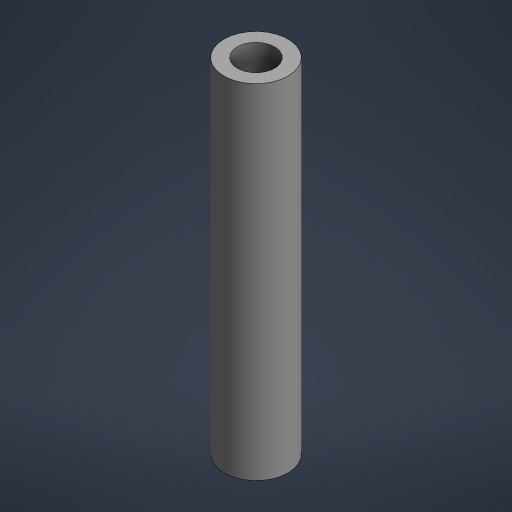
# Autodesk Inventor part: PDP_Spacer
Saved by Autodesk Inventor 2023 (Build 270158000, 158)
## iProperties
Part Number: PDP_Spacer
Material: Generic
Document SubType Name: Modeling
Designer: Conno
Mass: 1.96048 g
Surface Area: 21.8437 cm^2
Volume: 1.96048 cm^3
Density: 1 g/cm^3
Appearance: Default
Description: Spacer w/ clearance for 10-32 for PDP panel
DocNumber: PDP_Spacer.ipt
Folder: 2023\Swerve Electrical Concept\
VDS_Category: CAD
Author: Conno
Revision Number: A
Autodesk Inventor part; units mm, degrees
ref_plane "YZ Plane" through (0, 0, 0) normal (1, 0, 0) x (0, 1, 0)
ref_plane "XZ Plane" through (0, 0, 0) normal (0, 1, 0) x (-1, 0, 0)
ref_plane "XY Plane" through (0, 0, 0) normal (0, 0, 1) x (1, 0, 0)
sketch "Sketch1" plane through (0, 0, 0) normal (0, 1, 0) x (-1, 0, 0)
  circle A0 centre (0, 0) radius 2.5797
  circle A1 centre (0, 0) radius 4.445
  dimension "d0" = 5.1594
  dimension "d1" = 8.89
  constraints: 2 centre point, 2 coincident
  measures "d0" diameter of A0
  measures "d1" diameter of A1
extrude "Extrusion1" add sketch "Sketch1" along normal blind 47.625
body "Solid1"
